Autodesk Fusion 360 part; units mm, degrees
(part 2 of 2)
  constraint tangent A226 L211
  constraint tangent A231 L216
  constraint tangent A228 L213
  constraint tangent A230 L215
  constraint tangent A232 L217
  constraint tangent A233 L218
  constraint tangent A234 L219
  constraint tangent A235 L220
  constraint tangent L220 A236
  constraint tangent A236 L221
  constraint tangent A237 L222
  constraint tangent A239 L224
  constraint tangent A240 L225
  constraint concentric A6 A242
  constraint concentric A26 A243
  constraint concentric A24 A244
  constraint concentric A23 A245
  constraint concentric A21 A246
  constraint concentric A19 A247
  constraint concentric A16 A248
  constraint concentric A15 A249
  constraint concentric A14 A250
  constraint concentric A12 A251
  constraint concentric A11 A252
  constraint concentric A9 A253
  constraint concentric A8 A254
  constraint tangent A245 L231
  constraint tangent A243 L229
  constraint tangent A242 L227
  constraint tangent L229 A244
  constraint tangent A246 L233
  constraint tangent A250 L237
  constraint tangent A248 L235
  constraint tangent A249 L236
  constraint tangent A254 L242
  constraint tangent A252 L239
  constraint tangent A251 L243
  constraint tangent A252 L244
  constraint tangent A247 L247
  constraint tangent L245 A255
  constraint tangent L246 A255
  constraint tangent L246 A256
  constraint tangent L247 A256
  constraint tangent L243 A257
  constraint tangent L244 A257
  constraint tangent L237 A258
  constraint tangent L238 A258
  constraint tangent L239 A259
  constraint tangent L240 A259
  constraint tangent L226 A260
  constraint tangent L242 A260
  constraint tangent L227 A261
  constraint tangent L228 A261
  constraint tangent L231 A262
  constraint tangent L232 A262
  constraint tangent L233 A263
  constraint tangent L234 A263
  constraint coincident L206 L248.start
  constraint coincident L228 L248.end
  constraint perpendicular L228 L248
  constraint coincident L207 L249.start
  constraint coincident L229 L249.end
  constraint perpendicular L229 L249
  constraint tangent L250 A264
  constraint tangent L250 A265
  constraint tangent L251 A266
  constraint tangent L251 A267
  measures "d1" diameter of A0
  measures "d2" diameter of A1
  measures "d3" diameter of A2
  measures "d4" diameter of A3
  measures "d5" diameter of A4
  measures "d9" diameter of A111
  measures "d12" diameter of A112
  measures "d367" diameter of A210
  measures "d368" diameter of A211
  measures "d369" diameter of A212
  measures "d370" diameter of A213
  measures "d393" diameter of A214
  measures "d394" diameter of A215
extrude "Extrude1" add sketch "mriya-classic-fdm" along normal blind 10.5 contours L204 A220 L205 A221 L206 L207 A223 L208 A224 L209 A225 L210 A226 L211 A227 L212 A228 L213 A229 L214 A230 L215 A231 L216 A232 L217 A233 L218 A234 L219 A235 L220 A236 L221 A237 L222 A238 L223 A239 L224 A240 L225 A241 L226 A242 L227 L228 L229 A244 L230 A245 L231 L232 A246 L233 L234 A247 A248 L235 A249 L236 A250 L237 L238 A251 A252 L239 L240 A253 L241 A254 L242 L243 L244 L245 L246 L247 A255 A256 A257 A258 A259 A260 A261 A262 A263 L248 L249 makes body 1
extrude "Extrude2" add sketch "mriya-classic-fdm" along normal blind 17 contours L206 A222 L207 L228 A243 L229 L248 L249 bodies 1
extrude "Extrude3" add sketch "mriya-classic-fdm" along normal blind 3.7 contours A114 | A115 | A116 | A117 | A214 | A215 | L204 A220 L205 A221 L206 A222 L207 A223 L208 A224 L209 A225 L210 A226 L211 A227 L212 A228 L213 A229 L214 A230 L215 A231 L216 A232 L217 A233 L218 A234 L219 A235 L220 A236 L221 A237 L222 A238 L223 A239 L224 A240 L225 A241 L250 A264 A265 L251 A266 A267 | L206 L250 A264 A265 | L207 L251 A266 A267 bodies 1
extrude "Extrude13" add sketch "mriya-classic-fdm" along normal blind 1.8 contours A2 | L108 L109 A118 A119 A120 L182 L183 A216 | A121 L110 A122 L111 A123 L177 L178 A217 | A124 L112 A125 L113 A126 L114 A127 L115 | A128 L116 A129 L117 A130 L118 A131 L119 | A132 L120 A133 A134 L121 L184 L185 L186 A198 A199 | A135 L122 A136 A137 L123 L179 L180 L181 A200 A201 | A138 L124 A139 L125 A140 L126 A141 L127 | A142 L128 A143 L129 A144 L130 A145 L131 | A146 L132 A147 L133 A148 L134 A149 L135 | A150 L136 A151 L137 A152 L138 A153 L139 | A154 L140 A155 L141 A156 L142 A157 L143 | A158 L144 A159 L145 A160 L146 A161 L147 | A162 L148 A163 L149 A164 L150 A165 L151 | A166 L152 A167 L153 A168 L189 L190 L191 A202 A203 | A169 L154 A170 L155 A171 L156 A172 L157 | A173 L158 A174 L159 A175 L194 L195 L196 A204 A205 | A176 L160 A177 L161 A178 L162 A179 L163 | A180 A181 L164 A182 L165 L192 L193 A219 | A183 L166 A184 L167 A185 L168 A186 L169 | A187 A188 L170 A189 L171 L187 L188 A218 | A190 L172 A191 L173 A192 L174 A193 L175 | A194 L176 A195 L197 L198 L201 A206 A207 | A196 A197 L199 L200 A208 A209 L202 L203 bodies 1
extrude "Extrude14" add sketch "mriya-classic-fdm" along normal blind 2.7 contours A0 | A1 | A3 | A4 bodies 1
extrude "Extrude6" add sketch "mriya-classic-fdm" along normal blind 1.2 from surface at 14.1 contours L206 L250 A264 A265 bodies 1
extrude "Extrude12" add sketch "mriya-classic-fdm" along normal blind 1.2 from surface at 7.5 contours L207 L251 A266 A267 bodies 1
extrude "Extrude19" cut sketch "mriya-classic-fdm" along normal blind 1 from surface at 2.7 contours A214 | A215 bodies 1
chamfer "Chamfer24" distance 0.7 angle 45 2 edges at (-6.88, 9.5932, 7.5) (-16.4, 78.2132, 14.1) on bodies 1
sketch "power switch" plane through (-4.28, 0, 0) normal (1, 0, 0) x (0, 1, 0)
  line L0 (24.0932, 4.5) -> (24.0932, 9.2)
  line L1 (37.2932, 4.1) -> (24.4932, 4.1)
  arc A0 (37.6932, 9.2) -> (37.2932, 9.6) centre (37.2932, 9.2) ccw
  line L2 (36.0932, 8.3) -> (36.0932, 5.4)
  line L3 (25.6932, 8.3) -> (36.0932, 8.3)
  line L4 (36.0932, 5.4) -> (25.6932, 5.4)
  line L5 (25.6932, 5.4) -> (25.6932, 8.3)
  line L6 (24.4932, 9.6) -> (37.2932, 9.6)
  arc A1 (24.0932, 4.5) -> (24.4932, 4.1) centre (24.4932, 4.5) ccw
  arc A2 (37.2932, 4.1) -> (37.6932, 4.5) centre (37.2932, 4.5) ccw
  line L7 (37.6932, 9.2) -> (37.6932, 4.5)
  arc A3 (24.4932, 9.6) -> (24.0932, 9.2) centre (24.4932, 9.2) ccw
  line L8 (1.9932, 0) -> (76.4932, 0)
  line L9 (76.4932, 0) -> (76.4932, 17)
  line L10 (76.4932, 17) -> (19.3932, 17)
  line L11 (19.3932, 17) -> (19.3932, 10.5)
  line L12 (19.3932, 10.5) -> (1.9932, 10.5)
  line L13 (1.9932, 10.5) -> (1.9932, 0)
  constraint perpendicular L4 L5
  constraint vertical L5
  constraint perpendicular L3 L5
  constraint vertical L2
  constraint tangent A0 L6
  constraint tangent A0 L7
  constraint tangent A2 L7
  constraint tangent L1 A2
  constraint tangent L1 A1
  constraint tangent L0 A1
  constraint tangent L0 A3
  constraint tangent L6 A3
extrude "Extrude8" cut sketch "power switch" against normal blind 2.6 contours L2 L3 L4 L5 bodies 1
extrude "Extrude9" cut sketch "power switch" against normal blind 1.2 contours L0 L1 A0 L6 A1 A2 L7 A3 bodies 1
chamfer "Chamfer25" distance 1.43 angle 40 8 edges at (-4.28, 30.8932, 4.1) (-4.28, 24.2104, 4.2172) (-4.28, 24.0932, 6.85) (-4.28, 24.2104, 9.4828) (-4.28, 30.8932, 9.6) (-4.28, 37.576, 9.4828) (-4.28, 37.6932, 6.85) (-4.28, 37.576, 4.2172) measured on face at (-4.28, 63.5599, 8.7333) measured on face at (-4.28, 63.5599, 8.7333) measured on face at (-4.28, 63.5599, 8.7333) measured on face at (-4.28, 63.5599, 8.7333) measured on face at (-4.28, 63.5599, 8.7333) measured on face at (-4.28, 63.5599, 8.7333) measured on face at (-4.28, 63.5599, 8.7333) measured on face at (-4.28, 63.5599, 8.7333) on bodies 1
sketch "usb-c" plane through (0, 80.8132, 0) normal (0, 1, 0) x (-1, 0, 0)
  line L0 (19.8002, 8.8) -> (13.0003, 8.8)
  line L1 (21.8003, 13) -> (21.8003, 8.2)
  line L2 (21.0002, 11.2) -> (21.0002, 10)
  arc A0 (11.4003, 13.4) -> (11.0003, 13) centre (11.4003, 13) ccw
  arc A1 (21.4002, 7.8) -> (21.8002, 8.2) centre (21.4002, 8.2) ccw
  line L3 (11.8003, 10) -> (11.8003, 11.2)
  line L4 (21.4002, 7.8) -> (11.4002, 7.8)
  line L5 (11.4003, 13.4) -> (21.4002, 13.4)
  line L6 (13.0003, 12.4) -> (19.8002, 12.4)
  arc A2 (21.8002, 13) -> (21.4002, 13.4) centre (21.4002, 13) ccw
  arc A3 (11.0002, 8.2) -> (11.4002, 7.8) centre (11.4002, 8.2) ccw
  line L7 (11.0002, 8.2) -> (11.0002, 13)
  line L8 (8.6, 0) -> (41.0177, 0)
  line L9 (41.0177, 0) -> (41.0177, 10.5)
  line L10 (41.0177, 10.5) -> (25.7, 10.5)
  line L11 (25.7, 10.5) -> (25.7, 17)
  line L12 (25.7, 17) -> (8.6, 17)
  line L13 (8.6, 17) -> (8.6, 0)
  arc A4 (13.0003, 12.4) -> (11.8003, 11.2) centre (13.0003, 11.2) ccw
  arc A5 (21.0002, 11.2) -> (19.8002, 12.4) centre (19.8002, 11.2) ccw
  arc A6 (11.8003, 10) -> (13.0003, 8.8) centre (13.0003, 10) ccw
  arc A7 (19.8002, 8.8) -> (21.0002, 10) centre (19.8002, 10) ccw
  constraint perpendicular L1 L5
  constraint perpendicular L4 L7
  constraint horizontal L4
  constraint perpendicular L1 L4
  constraint tangent A0 L5
  constraint tangent A0 L7
  constraint tangent L5 A2
  constraint tangent L1 A2
  constraint tangent A3 L7
  constraint tangent L4 A3
  constraint tangent A1 L4
  constraint tangent L1 A1
  constraint tangent L6 A4
  constraint tangent L3 A4
  constraint tangent L6 A5
  constraint tangent L2 A5
  constraint tangent L0 A6
  constraint tangent L3 A6
  constraint tangent L2 A7
  constraint tangent L0 A7
extrude "Extrude17" cut sketch "usb-c" against normal blind 2.6 contours L0 L2 L3 L6 A4 A5 A6 A7 bodies 1
extrude "Extrude18" cut sketch "usb-c" against normal blind 1.2 contours L1 A0 A1 L4 L5 A2 A3 L7 bodies 1
chamfer "Chamfer26" distance 1.2 angle 45 8 edges at (-21.8003, 80.8132, 10.6) (-21.6831, 80.8132, 7.9172) (-16.4003, 80.8132, 7.8) (-11.1174, 80.8132, 7.9172) (-11.0003, 80.8132, 10.6) (-11.1174, 80.8132, 13.2828) (-16.4003, 80.8132, 13.4) (-21.6831, 80.8132, 13.2828) measured on face at (-23.6958, 80.8132, 2.602) measured on face at (-23.6958, 80.8132, 2.602) measured on face at (-23.6958, 80.8132, 2.602) measured on face at (-23.6958, 80.8132, 2.602) measured on face at (-23.6958, 80.8132, 2.602) measured on face at (-23.6958, 80.8132, 2.602) measured on face at (-23.6958, 80.8132, 2.602) measured on face at (-23.6958, 80.8132, 2.602) on bodies 1
chamfer "Chamfer27" distance 1 angle 45 87 edges at (-16.8358, -2.3268, 10.5) (-5.5453, -1.0615, 10.5) (-4.28, 10.6932, 10.5) (-33.3589, 80.8132, 10.5) (-41.4004, 80.8893, 10.5) (-42.0225, 81.4038, 10.5) (-43.8839, 82.7463, 10.5) (-51.773, 83.1132, 10.5) (-58.2004, 83.1893, 10.5) (-59.9225, 84.8038, 10.5) (-62.8839, 87.2463, 10.5) (-73.4, 87.6132, 10.5) (-83.9161, 87.2463, 10.5) (-86.3775, 85.3038, 10.5) (-87.5996, 84.1893, 10.5) (-94.5269, 84.1132, 10.5) (-102.9161, 83.7463, 10.5) (-107.4811, 79.7002, 10.5) (-111.1311, 76.2654, 10.5) (-115.9841, 76.1132, 10.5) (-121.9161, 75.7463, 10.5) (-123.7775, 74.4038, 10.5) (-124.3996, 73.8893, 10.5) (-131.4411, 73.8132, 10.5) (-141.1547, 72.5479, 10.5) (-142.42, 42.8932, 10.5) (-141.1547, 13.2385, 10.5) (-120.6213, 11.9732, 10.5) (-100.9154, 12.4162, 10.5) (-96.1725, 16.5326, 10.5) (-92.6689, 19.821, 10.5) (-84.6, 19.9732, 10.5) (-75.7843, 19.5642, 10.5) (-70.8069, 11.5856, 10.5) (-65.1622, 2.9302, 10.5) (-55.7575, 2.2732, 10.5) (-48.3996, 2.1971, 10.5) (-47.7775, 1.6826, 10.5) (-45.9161, 0.3401, 10.5) (-36.927, -0.0268, 10.5) (-29.3996, -0.1029, 10.5) (-28.7775, -0.6174, 10.5) (-26.9161, -1.9599, 10.5) (-16.8358, -2.3268, 0) (-26.9161, -1.9599, 0) (-28.7775, -0.6174, 0) (-29.3996, -0.1029, 0) (-36.927, -0.0268, 0) (-45.9161, 0.3401, 0) (-47.7775, 1.6826, 0) (-48.3996, 2.1971, 0) (-55.7575, 2.2732, 0) (-65.1622, 2.9302, 0) (-70.8069, 11.5856, 0) (-75.7843, 19.5642, 0) (-84.6, 19.9732, 0) (-92.6689, 19.821, 0) (-96.1725, 16.5326, 0) (-100.9154, 12.4162, 0) (-120.6213, 11.9732, 0) (-141.1547, 13.2385, 0) (-142.42, 42.8932, 0) (-141.1547, 72.5479, 0) (-131.4411, 73.8132, 0) (-124.3996, 73.8893, 0) (-123.7775, 74.4038, 0) (-121.9161, 75.7463, 0) (-115.9841, 76.1132, 0) (-111.1311, 76.2654, 0) (-107.4811, 79.7002, 0) (-102.9161, 83.7463, 0) (-94.5269, 84.1132, 0) (-87.5996, 84.1893, 0) (-86.3775, 85.3038, 0) (-83.9161, 87.2463, 0) (-73.4, 87.6132, 0) (-62.8839, 87.2463, 0) (-59.9225, 84.8038, 0) (-58.2004, 83.1893, 0) (-51.773, 83.1132, 0) (-43.8839, 82.7463, 0) (-42.0225, 81.4038, 0) (-41.4004, 80.8893, 0) (-24.8089, 80.8132, 0) (-5.5453, 79.5479, 0) (-4.28, 39.2432, 0) (-5.5453, -1.0615, 0) measured on face at (-140.6867, 34.0265, 10.5) measured on face at (-140.6867, 34.0265, 10.5) measured on face at (-140.6867, 34.0265, 10.5) measured on face at (-140.6867, 34.0265, 10.5) measured on face at (-140.6867, 34.0265, 10.5) measured on face at (-140.6867, 34.0265, 10.5) measured on face at (-140.6867, 34.0265, 10.5) measured on face at (-140.6867, 34.0265, 10.5) measured on face at (-140.6867, 34.0265, 10.5) measured on face at (-140.6867, 34.0265, 10.5) measured on face at (-140.6867, 34.0265, 10.5) measured on face at (-140.6867, 34.0265, 10.5) measured on face at (-140.6867, 34.0265, 10.5) measured on face at (-140.6867, 34.0265, 10.5) measured on face at (-140.6867, 34.0265, 10.5) measured on face at (-140.6867, 34.0265, 10.5) measured on face at (-140.6867, 34.0265, 10.5) measured on face at (-140.6867, 34.0265, 10.5) measured on face at (-140.6867, 34.0265, 10.5) measured on face at (-140.6867, 34.0265, 10.5) measured on face at (-140.6867, 34.0265, 10.5) measured on face at (-140.6867, 34.0265, 10.5) measured on face at (-140.6867, 34.0265, 10.5) measured on face at (-140.6867, 34.0265, 10.5) measured on face at (-140.6867, 34.0265, 10.5) measured on face at (-140.6867, 34.0265, 10.5) measured on face at (-140.6867, 34.0265, 10.5) measured on face at (-140.6867, 34.0265, 10.5) measured on face at (-140.6867, 34.0265, 10.5) measured on face at (-140.6867, 34.0265, 10.5) measured on face at (-140.6867, 34.0265, 10.5) measured on face at (-140.6867, 34.0265, 10.5) measured on face at (-140.6867, 34.0265, 10.5) measured on face at (-140.6867, 34.0265, 10.5) measured on face at (-140.6867, 34.0265, 10.5) measured on face at (-140.6867, 34.0265, 10.5) measured on face at (-140.6867, 34.0265, 10.5) measured on face at (-140.6867, 34.0265, 10.5) measured on face at (-140.6867, 34.0265, 10.5) measured on face at (-140.6867, 34.0265, 10.5) measured on face at (-140.6867, 34.0265, 10.5) measured on face at (-140.6867, 34.0265, 10.5) measured on face at (-140.6867, 34.0265, 10.5) measured on face at (-70.3411, 54.7799, 0) measured on face at (-25.9086, -2.2536, 7) measured on face at (-70.3411, 54.7799, 0) measured on face at (-70.3411, 54.7799, 0) measured on face at (-39.3085, -0.0268, 7) measured on face at (-44.4917, -0.0084, 7) measured on face at (-70.3411, 54.7799, 0) measured on face at (-70.3411, 54.7799, 0) measured on face at (-70.3411, 54.7799, 0) measured on face at (-64.7868, 2.7327, 7) measured on face at (-72.0994, 13.8733, 3.5) measured on face at (-70.3411, 54.7799, 0) measured on face at (-87.0345, 19.9732, 3.5) measured on face at (-70.3411, 54.7799, 0) measured on face at (-97.1241, 15.5811, 3.5) measured on face at (-100.4552, 12.6308, 7) measured on face at (-126.4475, 11.9732, 7) measured on face at (-140.6058, 12.7742, 7) measured on face at (-142.42, 51.7599, 3.5) measured on face at (-142.3419, 70.3108, 7) measured on face at (-70.3411, 54.7799, 0) measured on face at (-70.3411, 54.7799, 0) measured on face at (-70.3411, 54.7799, 0) measured on face at (-122.1086, 75.6616, 7) measured on face at (-70.3411, 54.7799, 0) measured on face at (-70.3411, 54.7799, 0) measured on face at (-70.3411, 54.7799, 0) measured on face at (-102.521, 83.8901, 7) measured on face at (-70.3411, 54.7799, 0) measured on face at (-70.3411, 54.7799, 0) measured on face at (-86.0783, 85.603, 3.5) measured on face at (-83.1148, 87.4989, 7) measured on face at (-70.3411, 54.7799, 0) measured on face at (-63.8914, 87.54, 7) measured on face at (-70.3411, 54.7799, 0) measured on face at (-70.3411, 54.7799, 0) measured on face at (-70.3411, 54.7799, 0) measured on face at (-42.4721, 81.8469, 3.5) measured on face at (-41.9233, 81.3045, 3.5) measured on face at (-70.3411, 54.7799, 0) measured on face at (-70.3411, 54.7799, 0) measured on face at (-4.4018, 77.5117, 11.3333) measured on face at (-4.28, 64.0364, 8.7333) measured on face at (-6.6205, -1.8466, 7) on bodies 1
fillet "Fillet30" radius 1.2 2 edges at (-4.28, 19.3932, 13.25) (-25.7, 80.8132, 13.25) on bodies 1
chamfer "Chamfer28" distance 1 angle 45 7 edges at (-4.28, 48.5432, 17) (-5.5453, 79.5479, 17) (-16.55, 80.8132, 17) (-25.3485, 80.4617, 17) (-25.7, 78.9132, 17) (-6.18, 19.3932, 17) (-4.6315, 19.7447, 17) measured on face at (-6.0133, 38.8265, 17) measured on face at (-6.0133, 38.8265, 17) measured on face at (-6.0133, 38.8265, 17) measured on face at (-24.5991, 80.8091, 14.5022) measured on face at (-6.0133, 38.8265, 17) measured on face at (-6.0133, 38.8265, 17) measured on face at (-4.2841, 20.4941, 14.5022) on bodies 1
chamfer "Chamfer20" distance 1 angle 45 6 edges at (-11.1722, 22.9091, 0) (-23.6722, 22.9091, 0) (-45.9722, 22.9591, 0) (-45.9722, 60.9591, 0) (-121.9722, 34.9591, 0) (-121.9722, 53.9591, 0) on bodies 1
sketch "silicone feets" plane through (0, 0, 0) normal (0, 0, -1) x (1, 0, 0)
  circle A0 centre (-120.9, -34.5432) radius 2.15
  circle A1 centre (-44.9, -22.5432) radius 2.15
  circle A2 centre (-10.1, -22.4932) radius 2.15
  circle A3 centre (-22.6, -22.4932) radius 2.15
  circle A4 centre (-44.9, -60.5432) radius 2.15
  circle A5 centre (-120.9, -53.5432) radius 2.15
  circle A6 centre (-11.78, -73.3132) radius 4.1
  circle A7 centre (-73.4, -80.1132) radius 4.1
  circle A8 centre (-134.92, -66.3132) radius 4.1
  circle A9 centre (-134.92, -19.4732) radius 4.1
  circle A10 centre (-61.1688, -9.7732) radius 4.1
  circle A11 centre (-11.78, -5.1732) radius 4.1
  line L0 (-8.6, 1.3268) -> (-25.0716, 1.3268)
  arc A12 (-25.0716, 1.3268) -> (-27.7727, 0.2079) centre (-25.0715, -2.4933) ccw
  line L1 (-27.7727, 0.2079) -> (-28.3681, -0.3874)
  arc A13 (-29.7823, -0.9732) -> (-28.3681, -0.3874) centre (-29.7823, 1.0268) ccw
  line L2 (-29.7823, -0.9732) -> (-44.0716, -0.9732)
  arc A14 (-44.0716, -0.9732) -> (-46.7727, -2.0921) centre (-44.0715, -4.7933) ccw
  line L3 (-46.7727, -2.0921) -> (-47.3681, -2.6874)
  arc A15 (-48.7823, -3.2732) -> (-47.3681, -2.6874) centre (-48.7823, -1.2732) ccw
  line L4 (-48.7823, -3.2732) -> (-62.7328, -3.2732)
  arc A16 (-62.7328, -3.2732) -> (-66.0587, -5.2142) centre (-62.7328, -7.0932) ccw
  line L5 (-66.0587, -5.2142) -> (-73.8138, -18.9408)
  arc A17 (-77.2964, -20.9732) -> (-73.8138, -18.9408) centre (-77.2964, -16.9732) ccw
  line L6 (-77.2964, -20.9732) -> (-91.9035, -20.9732)
  arc A18 (-94.0248, -20.0945) -> (-91.9035, -20.9732) centre (-91.9035, -17.9732) ccw
  line L7 (-94.0248, -20.0945) -> (-99.7343, -14.385)
  arc A19 (-99.7344, -14.385) -> (-103.1426, -12.9732) centre (-103.1426, -17.7931) ccw
  line L8 (-103.1426, -12.9732) -> (-138.1, -12.9732)
  arc A20 (-138.1, -12.9732) -> (-141.42, -16.2932) centre (-138.1, -16.2932) ccw
  line L9 (-141.42, -16.2932) -> (-141.42, -69.4932)
  arc A21 (-141.42, -69.4932) -> (-138.1, -72.8132) centre (-138.1, -69.4932) ccw
  line L10 (-138.1, -72.8132) -> (-124.7823, -72.8132)
  arc A22 (-123.3681, -73.399) -> (-124.7823, -72.8132) centre (-124.7823, -74.8132) ccw
  line L11 (-123.3681, -73.399) -> (-122.7728, -73.9943)
  arc A23 (-122.7727, -73.9943) -> (-120.0716, -75.1132) centre (-120.0716, -71.2933) ccw
  line L12 (-120.0716, -75.1132) -> (-111.8965, -75.1132)
  arc A24 (-109.7752, -75.9919) -> (-111.8965, -75.1132) centre (-111.8965, -78.1132) ccw
  line L13 (-109.7752, -75.9919) -> (-103.7727, -81.9944)
  arc A25 (-103.7727, -81.9944) -> (-101.0716, -83.1132) centre (-101.0716, -79.2933) ccw
  line L14 (-101.0716, -83.1132) -> (-87.9823, -83.1132)
  arc A26 (-86.5681, -83.699) -> (-87.9823, -83.1132) centre (-87.9823, -85.1132) ccw
  line L15 (-86.5681, -83.699) -> (-84.7728, -85.4943)
  arc A27 (-84.7727, -85.4943) -> (-82.0716, -86.6132) centre (-82.0716, -82.7933) ccw
  line L16 (-82.0716, -86.6132) -> (-64.7284, -86.6132)
  arc A28 (-64.7284, -86.6132) -> (-62.0273, -85.4943) centre (-64.7285, -82.7931) ccw
  line L17 (-62.0273, -85.4943) -> (-59.2319, -82.699)
  arc A29 (-57.8177, -82.1132) -> (-59.2319, -82.699) centre (-57.8177, -84.1132) ccw
  line L18 (-57.8177, -82.1132) -> (-45.7284, -82.1132)
  arc A30 (-45.7284, -82.1132) -> (-43.0273, -80.9943) centre (-45.7285, -78.2931) ccw
  line L19 (-43.0273, -80.9943) -> (-42.4319, -80.399)
  arc A31 (-41.0177, -79.8132) -> (-42.4319, -80.399) centre (-41.0177, -81.8132) ccw
  line L20 (-41.0177, -79.8132) -> (-8.6, -79.8132)
  arc A32 (-8.6, -79.8132) -> (-5.28, -76.4932) centre (-8.6, -76.4932) ccw
  line L21 (-5.28, -76.4932) -> (-5.28, -1.9932)
  arc A33 (-5.28, -1.9932) -> (-8.6, 1.3268) centre (-8.6, -1.9932) ccw
  dimension "d374" = 8.2
  dimension "d375" = 8.2
  dimension "d376" = 8.2
  dimension "d377" = 8.2
  dimension "d378" = 8.2
  dimension "d379" = 8.2
  dimension "d476" = 6.5
  dimension "d477" = 6.5
  dimension "d478" = 6.5
  dimension "d479" = 6.5
  dimension "d480" = 6.5
  dimension "d481" = 6.5
  dimension "d482" = 6.5
  dimension "d483" = 6.5
  dimension "d484" = 6.5
  dimension "d485" = 6.5
  dimension "d486" = 6.5
  measures "d374" diameter of A6
  measures "d375" diameter of A7
  measures "d376" diameter of A8
  measures "d377" diameter of A9
  measures "d378" diameter of A10
  measures "d379" diameter of A11
  measures "d476" distance of A6.centre L21
  measures "d477" distance of A6.centre L20
  measures "d478" distance of A7.centre L16
  measures "d479" distance of A8.centre L9
  measures "d480" distance of A8.centre L10
  measures "d481" distance of A9.centre L9
  measures "d482" distance of A9.centre L8
  measures "d483" distance of A10.centre L5
  measures "d484" distance of A10.centre L4
  measures "d485" distance of A11.centre L0
  measures "d486" distance of A11.centre L21
extrude "Extrude15" cut sketch "silicone feets" against normal blind 0.9 contours A6 | A7 | A8 | A9 | A10 | A11 bodies 1
mirror "Mirror1" about plane through (0, 0, 0) normal (1, 0, 0) of bodies 1 makes body 2
named bodies: "Left", "Right"
